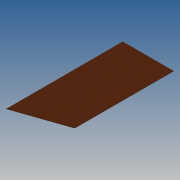
# Autodesk Inventor part: roof2
Saved by Autodesk Inventor 2013 (Build 170138000, 138)
## iProperties
Created: 2013-08-10
Part Number: roof2
Material: Wood (Walnut)
Document SubType Name: Modeling
Designer: ddeboer
Mass: 60927.1 g
Surface Area: 176058 cm^2
Volume: 110777 cm^3
Density: 0.55 g/cm^3
Author: ddeboer
Autodesk Inventor part; units mm, degrees
ref_plane "YZ Plane" through (0, 0, 0) normal (1, 0, 0) x (0, 1, 0)
ref_plane "XZ Plane" through (0, 0, 0) normal (0, 1, 0) x (-1, 0, 0)
ref_plane "XY Plane" through (0, 0, 0) normal (0, 0, 1) x (1, 0, 0)
sketch "Sketch1" plane through (0, 0, 0) normal (0, 1, 0) x (-1, 0, 0)
  line L0 (-2209.8, 0) -> (-2209.8, -4292.6)
  line L1 (-2209.8, -4292.6) -> (0, -4292.6)
  line L2 (0, -4292.6) -> (0, 0)
  line L3 (0, 0) -> (0, 762)
  line L4 (0, 762) -> (-2209.8, 0)
  dimension "d0" = 2209.8
  dimension "d1" = 4292.6
  dimension "d4" = 762
  constraints: 10 end point, 1 collinear, 1 parallel
  measures "d0" distance of L2.end L0.start
  measures "d1" distance of L1.end L2.end
  measures "d4" distance of L2.end L3.end
extrude "Extrusion1" add sketch "Sketch1" along normal blind 12.7
body "Solid1"
